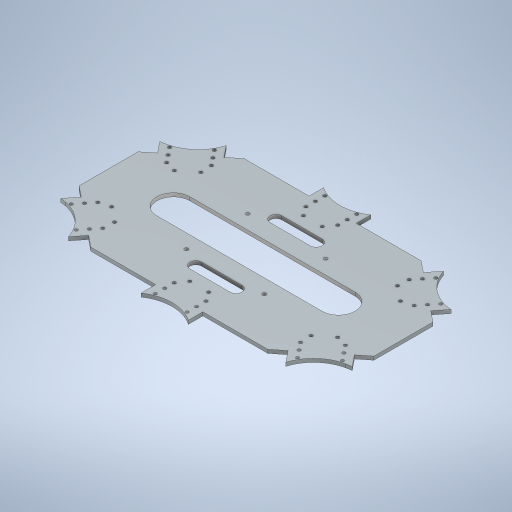
# Autodesk Inventor part: base
Saved by Autodesk Inventor 2024 (Build 280153000, 153)
## iProperties
Created: 2024-03-15
Part Number: base
Material: Generic
Document SubType Name: Modeling
Designer: kamil
Density: 1 g/cm^3
Appearance: Default
Author: kamil
Autodesk Inventor part; units mm, degrees
ref_plane "YZ Plane" through (0, 0, 0) normal (1, 0, 0) x (0, 1, 0)
ref_plane "XZ Plane" through (0, 0, 0) normal (0, 1, 0) x (-1, 0, 0)
ref_plane "XY Plane" through (0, 0, 0) normal (0, 0, 1) x (1, 0, 0)
sketch "Sketch1" plane through (0, 0, 0) normal (0, 1, 0) x (-1, 0, 0)
  line L0 (125, 65) -> (-125, 65)
  line L1 (-125, 65) -> (-125, -65)
  line L2 (-125, -65) -> (125, -65)
  line L3 (125, -65) -> (125, 65)
  line L4 (125, -65) -> (-125, 65) construction
  line L5 (125, 65) -> (-125, -65) construction
  line L6 (16, 65) -> (-16, 65)
  line L7 (-16, 65) -> (-16, 75)
  line L8 (16, 75) -> (16, 65)
  circle A0 centre (13.5, 55.845) radius 1.325
  circle A1 centre (-13.5, 55.845) radius 1.325
  circle A2 centre (8, 48.1625) radius 1.325
  circle A3 centre (-8, 48.1625) radius 1.325
  circle A4 centre (13.5, 63.845) radius 1.325
  circle A5 centre (-13.5, 63.845) radius 1.325
  circle A6 centre (13.5, 71.845) radius 1.325
  circle A7 centre (-13.5, 71.845) radius 1.325
  arc A8 (-16, 75) -> (16, 75) centre (0, 106.8224) ccw
  line L9 (125, 0) -> (-125, 0) construction
  line L10 (-125, -25) -> (-75, -65)
  line L11 (0, -65) -> (0, 65) construction
  line L12 (-125, 25) -> (-75, 65)
  line L13 (125, -25) -> (75, -65)
  line L14 (125, 25) -> (75, 65)
  line L15 (-16, -65) -> (-16, -75)
  line L16 (16, -75) -> (16, -65)
  circle A9 centre (13.5, -55.845) radius 1.325
  circle A10 centre (-13.5, -55.845) radius 1.325
  circle A11 centre (8, -48.1625) radius 1.325
  circle A12 centre (-8, -48.1625) radius 1.325
  circle A13 centre (13.5, -63.845) radius 1.325
  circle A14 centre (-13.5, -63.845) radius 1.325
  circle A15 centre (13.5, -71.845) radius 1.325
  circle A16 centre (-13.5, -71.845) radius 1.325
  arc A17 (16, -75) -> (-16, -75) centre (0, -106.8224) ccw
  circle A18 centre (-83.3378, -36.5977) radius 1.325
  circle A19 centre (-83.8422, -46.0325) radius 1.325
  circle A20 centre (-88.8398, -52.2795) radius 1.325
  circle A21 centre (-93.8374, -58.5264) radius 1.325
  arc A22 (-93.8562, -62.5518) -> (-118.8439, -42.5615) centre (-126.2293, -77.4056) ccw
  circle A23 centre (-114.9208, -41.6596) radius 1.325
  circle A24 centre (-109.9232, -35.4126) radius 1.325
  circle A25 centre (-104.9256, -29.1657) radius 1.325
  circle A26 centre (-95.8316, -26.6025) radius 1.325
  line L17 (-83.3378, -36.5977) -> (-95.8316, -26.6025) construction
  line L18 (-88.8398, -52.2795) -> (-109.9232, -35.4126) construction
  line L19 (-89.5847, -31.6001) -> (-99.3815, -43.846) construction
  line L20 (-83.8422, -46.0325) -> (-104.9256, -29.1657) construction
  line L21 (-93.8374, -58.5264) -> (-114.9208, -41.6596) construction
  line L22 (-99.3815, -43.846) -> (-103.9787, -49.5925) construction
  line L23 (-104.3791, -50.093) -> (-103.9787, -49.5925) construction
  circle A27 centre (-83.3378, 36.5977) radius 1.325
  circle A28 centre (-83.8422, 46.0325) radius 1.325
  circle A29 centre (-88.8398, 52.2795) radius 1.325
  circle A30 centre (-93.8374, 58.5264) radius 1.325
  arc A31 (-118.8439, 42.5615) -> (-93.8562, 62.5518) centre (-126.2293, 77.4056) ccw
  circle A32 centre (-114.9208, 41.6596) radius 1.325
  circle A33 centre (-109.9232, 35.4126) radius 1.325
  circle A34 centre (-104.9256, 29.1657) radius 1.325
  circle A35 centre (-95.8316, 26.6025) radius 1.325
  line L24 (-83.3378, 36.5977) -> (-95.8316, 26.6025) construction
  line L25 (-88.8398, 52.2795) -> (-109.9232, 35.4126) construction
  line L26 (-89.5847, 31.6001) -> (-99.3815, 43.846) construction
  line L27 (-83.8422, 46.0325) -> (-104.9256, 29.1657) construction
  line L28 (-93.8374, 58.5264) -> (-114.9208, 41.6596) construction
  line L29 (-99.3815, 43.846) -> (-103.9787, 49.5925) construction
  line L30 (-104.3791, 50.093) -> (-103.9787, 49.5925) construction
  circle A36 centre (83.3378, -36.5977) radius 1.325
  circle A37 centre (83.8422, -46.0325) radius 1.325
  circle A38 centre (88.8398, -52.2795) radius 1.325
  circle A39 centre (93.8374, -58.5264) radius 1.325
  arc A40 (118.8439, -42.5615) -> (93.8562, -62.5518) centre (126.2293, -77.4056) ccw
  circle A41 centre (114.9208, -41.6596) radius 1.325
  circle A42 centre (109.9232, -35.4126) radius 1.325
  circle A43 centre (104.9256, -29.1657) radius 1.325
  circle A44 centre (95.8316, -26.6025) radius 1.325
  line L31 (83.3378, -36.5977) -> (95.8316, -26.6025) construction
  line L32 (88.8398, -52.2795) -> (109.9232, -35.4126) construction
  line L33 (83.8422, -46.0325) -> (104.9256, -29.1657) construction
  line L34 (93.8374, -58.5264) -> (114.9208, -41.6596) construction
  line L35 (99.3815, -43.846) -> (103.9787, -49.5925) construction
  line L36 (104.3791, -50.093) -> (103.9787, -49.5925) construction
  circle A45 centre (83.3378, 36.5977) radius 1.325
  circle A46 centre (95.8316, 26.6025) radius 1.325
  line L37 (83.3378, 36.5977) -> (95.8316, 26.6025) construction
  line L38 (89.5847, 31.6001) -> (99.3815, 43.846) construction
  line L39 (83.8422, 46.0325) -> (104.9256, 29.1657) construction
  line L40 (88.8398, 52.2795) -> (109.9232, 35.4126) construction
  line L41 (93.8374, 58.5264) -> (114.9208, 41.6596) construction
  line L42 (99.3815, 43.846) -> (103.9787, 49.5925) construction
  line L43 (104.3791, 50.093) -> (103.9787, 49.5925) construction
  arc A47 (93.8562, 62.5518) -> (118.8439, 42.5615) centre (126.2293, 77.4056) ccw
  circle A48 centre (114.9208, 41.6596) radius 1.325
  circle A49 centre (109.9232, 35.4126) radius 1.325
  circle A50 centre (104.9256, 29.1657) radius 1.325
  circle A51 centre (83.8422, 46.0325) radius 1.325
  circle A52 centre (88.8398, 52.2795) radius 1.325
  circle A53 centre (93.8374, 58.5264) radius 1.325
  line L44 (99.3815, -43.846) -> (89.5847, -31.6001) construction
  line L45 (93.8562, 62.5518) -> (87.6919, 54.8465)
  line L46 (118.8439, 42.5615) -> (112.6797, 34.8562)
  line L47 (118.8439, -42.5615) -> (112.6797, -34.8562)
  line L48 (93.8562, -62.5518) -> (87.6919, -54.8465)
  line L49 (-118.8439, -42.5615) -> (-112.6797, -34.8562)
  line L50 (-93.8562, -62.5518) -> (-87.6919, -54.8465)
  line L51 (-93.8562, 62.5518) -> (-87.6919, 54.8465)
  line L52 (-118.8439, 42.5615) -> (-112.6797, 34.8562)
  line L53 (-20, 65) -> (-20, 77.4056)
  arc A54 (-20.0262, 77.3671) -> (-16, 75) centre (0, 106.8224) ccw
  line L54 (0, 106.8224) -> (0, 65) construction
  line L55 (20, 65) -> (20, 77.4056)
  arc A55 (16, 75) -> (20.0262, 77.3671) centre (0, 106.8224) ccw
  line L56 (-20, -65) -> (-20, -77.4056)
  arc A56 (-16, -75) -> (-20.0262, -77.3671) centre (0, -106.8224) ccw
  line L57 (20, -65) -> (20, -77.4056)
  arc A57 (20.0262, -77.3671) -> (16, -75) centre (0, -106.8224) ccw
  arc A58 (-92.2003, -66.885) -> (-93.8562, -62.5518) centre (-126.2293, -77.4056) ccw
  line L58 (-92.2003, -66.885) -> (-84.5684, -57.3452)
  arc A59 (-118.8439, -42.5614) -> (-123.435, -41.8971) centre (-126.2294, -77.4056) ccw
  line L59 (-123.435, -41.8971) -> (-115.8031, -32.3574)
  arc A60 (-93.8562, 62.5518) -> (-92.2003, 66.885) centre (-126.2293, 77.4056) ccw
  line L60 (-92.2003, 66.885) -> (-84.5684, 57.3452)
  line L61 (-123.435, 41.8971) -> (-115.8031, 32.3574)
  arc A61 (-123.435, 41.8971) -> (-118.8439, 42.5614) centre (-126.2294, 77.4056) ccw
  arc A62 (93.8562, -62.5518) -> (92.2003, -66.885) centre (126.2293, -77.4056) ccw
  line L62 (92.2003, -66.885) -> (84.5684, -57.3452)
  line L63 (123.435, -41.8971) -> (115.8031, -32.3574)
  arc A63 (123.435, -41.8971) -> (118.8439, -42.5614) centre (126.2294, -77.4056) ccw
  line L64 (92.2003, 66.885) -> (84.5684, 57.3452)
  arc A64 (92.2003, 66.885) -> (93.8562, 62.5518) centre (126.2293, 77.4056) ccw
  line L65 (123.435, 41.8971) -> (115.8031, 32.3574)
  arc A65 (118.8439, 42.5614) -> (123.435, 41.8971) centre (126.2294, 77.4056) ccw
  line L66 (92.5, 0) -> (-92.5, 0) construction
  circle A66 centre (33, 26) radius 1.5
  circle A67 centre (33, -26) radius 1.5
  circle A68 centre (-33, 26) radius 1.5
  circle A69 centre (-33, -26) radius 1.5
  line L67 (84, 0) -> (-84, 0) construction
  line L68 (70, 14) -> (-70, 14)
  line L69 (-70, -14) -> (70, -14)
  arc A70 (70, -14) -> (70, 14) centre (70, 0) ccw
  arc A71 (-70, 14) -> (-70, -14) centre (-70, 0) ccw
  line L70 (22, -34) -> (-22, -34) construction
  line L71 (17, -39) -> (-17, -39)
  line L72 (-17, -29) -> (17, -29)
  arc A72 (17, -39) -> (17, -29) centre (17, -34) ccw
  arc A73 (-17, -29) -> (-17, -39) centre (-17, -34) ccw
  line L73 (17, 39) -> (-17, 39)
  line L74 (-17, 29) -> (17, 29)
  arc A74 (17, 29) -> (17, 39) centre (17, 34) ccw
  arc A75 (-17, 39) -> (-17, 29) centre (-17, 34) ccw
  point P0 (0, 0)
  point P1 (0, 0)
  point P2 (-16, 70)
  point P3 (115.8031, 32.3575)
  point P4 (118.8439, 42.5615)
  point P5 (118.8439, -42.5615)
  point P6 (115.8031, -32.3575)
  point P7 (-20, -77.3493)
  point P8 (20, -77.3493)
  point P9 (-118.8439, -42.5615)
  point P10 (-115.8031, -32.3575)
  point P11 (-118.8439, 42.5615)
  point P12 (-115.8031, 32.3575)
  point P13 (-20, 77.3493)
  point P14 (20, 77.3493)
  point P15 (0, 28)
  point P16 (0, 0)
  point P17 (0, 0)
  point P18 (0, -34)
  dimension "d0" = 250
  dimension "d1" = 130
  dimension "d2" = 32
  dimension "d4" = 2.65
  dimension "d5" = 2.65
  dimension "d6" = 2.65
  dimension "d7" = 2.65
  dimension "d8" = 16
  dimension "d9" = 5.5
  dimension "d10" = 5.5
  dimension "d11" = 2.5
  dimension "d12" = 2.5
  dimension "d13" = 2.65
  dimension "d14" = 2.65
  dimension "d15" = 2.65
  dimension "d16" = 2.65
  dimension "d18" = 8
  dimension "d19" = 8
  dimension "d20" = 8
  dimension "d21" = 8
  dimension "d22" = 25
  dimension "d23" = 50
  dimension "d28" = 13.5
  dimension "d29" = 4
  dimension "d41" = 3
  dimension "d42" = 26
  dimension "d43" = 33
  dimension "d44" = 28
  dimension "d45" = 55
  dimension "d46" = 55
  dimension "d47" = 34
  dimension "d48" = 108
  dimension "d49" = 108
  dimension "d50" = 5
  dimension "d51" = 2.65
  dimension "d52" = 2.65
  dimension "d53" = 2.65
  dimension "d54" = 2.65
  dimension "d55" = 2.65
  dimension "d56" = 2.65
  dimension "d57" = 2.65
  dimension "d58" = 2.65
  constraints: 156 end point, 107 symmetric about line, 76 centre point, 54 point on circle, 21 point on line, 14 midpoint, 13 perpendicular, 8 tangent, 5 parallel, 3 coincident, 3 horizontal, 2 collinear, 2 horizontal alignment, 51 other
  measures "d0" distance of L1.end L2.end
  measures "d1" distance of L0.end L1.end
  measures "d2" distance from line of point (-16, 70) L8
  measures "d4" diameter of A0
  measures "d5" diameter of A1
  measures "d6" diameter of A2
  measures "d7" diameter of A3
  measures "d8" distance of A3.centre A2.centre
  measures "d9" horizontal distance of A3.centre A1.centre
  measures "d10" horizontal distance of A2.centre A0.centre
  measures "d11" distance from line of A1.centre L7
  measures "d12" distance from line of L8 A0.centre
  measures "d13" diameter of A4
  measures "d14" diameter of A5
  measures "d15" diameter of A6
  measures "d16" diameter of A7
  measures "d18" distance of A4.centre A6.centre
  measures "d19" distance of A0.centre A4.centre
  measures "d20" distance of A7.centre A5.centre
  measures "d21" distance of A5.centre A1.centre
  measures "d22" distance from line of L9 L10.start
  measures "d23" distance of L1.end L10.end
  measures "d28" distance from line of L11 A0.centre
  measures "d29" distance between parallel lines of L53 L7
  measures "d41" diameter of A66
  measures "d42" distance from line of L66 A66.centre
  measures "d43" distance from line of L11 A66.centre
  measures "d44" diameter of A71
  measures "d45" distance from line of L3 A70.centre
  measures "d46" distance from line of L1 A71.centre
  measures "d47" distance from line of L67 A72.centre
  measures "d48" distance from line of L3 A72.centre
  measures "d49" distance from line of L1 A73.centre
  measures "d50" radius of A73
  measures "d51" diameter of A18
  measures "d52" diameter of A19
  measures "d53" diameter of A20
  measures "d54" diameter of A21
  measures "d55" diameter of A26
  measures "d56" diameter of A25
  measures "d57" diameter of A24
  measures "d58" diameter of A23
extrude "Extrusion1" add sketch "Sketch1" along normal blind 3 contours L14 A52 A49 L3 L13 A42 A38 L2 A13 A14 L10 A20 A24 L1 L12 A33 A29 L0 A5 A4 | L0 L8 A55 L55 | L64 A64 L0 | L0 A64 L45 L14 L64 | L0 A4 A5 L7 A8 L8 | L45 A47 L46 L14 A49 A52 | L7 L0 L53 A54 | A65 L65 L14 L46 | L63 A63 L47 L13 | A62 L62 L2 | L2 L62 L13 L48 A62 | L47 A40 L48 L13 A38 A42 | L60 L12 L51 A60 L0 | L0 A60 L60 | L12 A29 A33 L52 A31 L51 | L57 A57 L16 L2 | L52 L12 L61 A61 | L16 A17 L15 L2 A14 A13 | L10 L49 A59 L59 | A56 L56 L2 L15 | A58 L50 L10 L58 L2 | L2 L58 A58 | L10 A24 A20 L50 A22 L49
body "Solid1"
